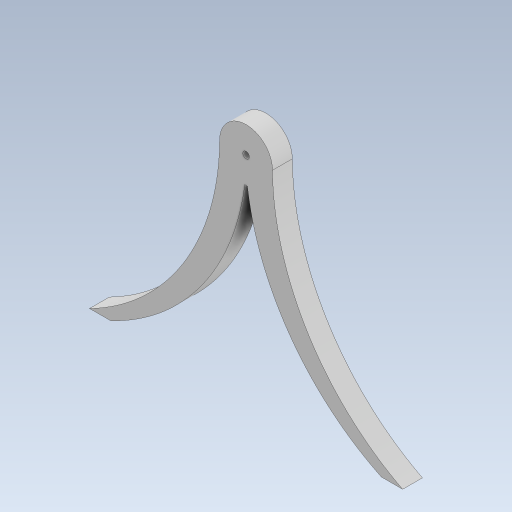
# Autodesk Inventor part: rod support main
Saved by Autodesk Inventor 2023 (Build 270158000, 158)
## iProperties
Created: 2023-03-23
Part Number: rod support main
Material: Generic
Document SubType Name: Modeling
Designer: dverd
Density: 1 g/cm^3
Appearance: Default
Author: dverd
Autodesk Inventor part; units mm, degrees
ref_plane "YZ Plane" through (0, 0, 0) normal (1, 0, 0) x (0, 1, 0)
ref_plane "XZ Plane" through (0, 0, 0) normal (0, 1, 0) x (-1, 0, 0)
ref_plane "XY Plane" through (0, 0, 0) normal (0, 0, 1) x (1, 0, 0)
sketch "Sketch1" plane through (0, 0, 0) normal (0, 0, 1) x (1, 0, 0)
  line L0 (0, 0) -> (203.2, 0)
  line L1 (203.2, 0) -> (203.2, -203.2)
  line L2 (0, -203.2) -> (0, 0)
  line L3 (0, -101.6) -> (203.2, -101.6)
  circle A0 centre (101.6, -101.6) radius 1.5635
  circle A1 centre (101.6, -101.6) radius 12.7
  arc A2 (26.281, -203.2) -> (88.9003, -101.509) centre (-26.321, -100.6834) ccw
  arc A3 (36.5054, -203.2) -> (101.6, -107.95) centre (-13.2987, -99.2953) ccw
  line L4 (101.6, -246.9942) -> (101.6, 0)
  arc A4 (114.2997, -101.509) -> (176.919, -203.2) centre (229.521, -100.6834) ccw
  arc A5 (101.6, -107.95) -> (166.6946, -203.2) centre (216.4987, -99.2953) ccw
  line L5 (166.6946, -203.2) -> (176.919, -203.2)
  line L6 (26.281, -203.2) -> (36.5054, -203.2)
  line L7 (0, -203.2) -> (203.2, -203.2)
  point P0 (88.9, -101.6)
  point P1 (88.8996, -101.6)
  point P2 (100.9466, -114.2832)
  point P3 (102.2534, -114.2832)
  point P4 (114.3004, -101.6)
  point P5 (114.3, -101.6)
  point P6 (171.8068, -203.2)
  point P7 (101.6, -123.4971)
  point P8 (114.2997, -101.509)
  dimension "d10" = 25.4
  dimension "d7" = 203.2
  dimension "d8" = 203.2
  dimension "d9" = 3.127
  dimension "d11" = 115.2242
  dimension "d12" = 115.2242
  dimension "d15" = 26.281
  dimension "d16" = 6.35
  dimension "d18" = 101.6
  dimension "d19" = 10.2243
  constraints: 16 end point, 8 point on circle, 6 midpoint, 5 centre point, 5 horizontal, 5 symmetric about line, 1 coincident, 1 parallel, 1 perpendicular, 1 vertical, 6 other
  measures "d7" distance of L1.end L2.start
  measures "d8" distance of L0.end L1.end
  measures "d9" diameter of A0
  measures "d11" radius of A2
  measures "d12" radius of A3
  measures "d15" distance of L2.start L6.start
  measures "d16" distance of point (101.6, -101.6) A3.end
  measures "d18" distance from line of A0.centre L5
  measures "d19" distance of L6.start L6.end
extrude "Extrusion1" add sketch "Sketch1" along normal blind 9.525 contours L4 A0 L3 A1 | A1 L3 A0 L4 | L3 A0 L4 A3 A1 | A1 A3 L6 A2 | A3 L4 A1 | A1 A5 L4 A0 L3 | A4 L5 A5 A1 | L4 A5 A1
body "Solid1"
